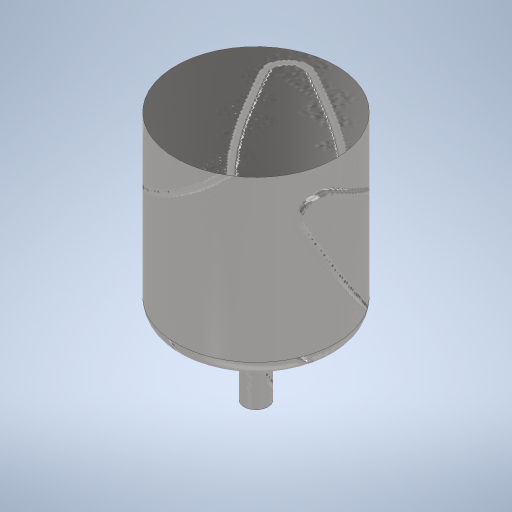
# Autodesk Inventor part: motor_ven
Saved by Autodesk Inventor 2023 (Build 270158000, 158)
## iProperties
Created: 2023-08-09
Part Number: motor_ven
Material: Genérico
Document SubType Name: Modeling
Designer: azeve
Density: 1 g/cm^3
Appearance: Padrão
Author: azeve
Autodesk Inventor part; units mm, degrees
ref_plane "YZ Plane" through (0, 0, 0) normal (1, 0, 0) x (0, 1, 0)
ref_plane "XZ Plane" through (0, 0, 0) normal (0, 1, 0) x (-1, 0, 0)
ref_plane "XY Plane" through (0, 0, 0) normal (0, 0, 1) x (1, 0, 0)
sketch "Esboço1" plane through (0, 0, 0) normal (0, 0, 1) x (1, 0, 0)
  line L0 (0, 0) -> (0, 22)
  line L1 (0, 22) -> (10, 22)
  line L2 (10, 22) -> (10, 19.8993)
  line L3 (10, 19.8993) -> (10, 0)
  line L4 (10, 0) -> (0, 0)
  line L5 (0, 0) -> (1.5, 0)
  line L6 (1.5, 0) -> (1.5, -9.13)
  line L7 (1.5, -9.13) -> (0, -9.13)
  line L8 (0, -9.13) -> (0, 0)
  line L9 (1.5, 0) -> (1.5, -1)
  line L10 (1.5, -1) -> (4.5, -1)
  line L11 (4.5, -1) -> (4.5, -6.8)
  line L12 (4.5, -6.8) -> (1.5, -6.8)
  line L13 (1.5, -6.8) -> (1.5, -1)
  line L14 (1.5, -6.8) -> (0, -6.8)
  line L15 (0, -1) -> (1.5, -1)
  line L16 (4.5, -1) -> (4.5, -3.025)
  line L17 (4.5, -3.025) -> (6.5557, -3.025)
  line L18 (6.5557, -3.025) -> (6.5557, -4.795)
  dimension "d0" = 22
  dimension "d1" = 10
  dimension "d2" = 1.5
  dimension "d4" = 9.13
  dimension "d7" = 1
  dimension "d8" = 3
  dimension "d9" = 5.8
  dimension "d10" = 2.025
  dimension "d11" = 1.77
  constraints: 38 end point, 8 point on line, 6 perpendicular, 5 vertical, 3 horizontal, 1 collinear
  measures "d0" distance of L0.start L0.end
  measures "d1" distance of L0.end L1.end
  measures "d2" distance of L0.start L5.end
  measures "d4" distance of L5.end L6.end
  measures "d7" distance of L5.end L9.end
  measures "d8" distance of L9.end L10.end
  measures "d9" distance of L10.end L11.end
  measures "d10" distance of L10.end L16.end
  measures "d11" distance of L17.end L18.end
revolve "Revolução1" add sketch "Esboço1" angle 360 about axis through (0, 0, 0) along (0, 1, 0) contours L0 L1 L2 L3 L4 | L4 L6 L15 L8 | L15 L6 L14 L8 | L14 L6 L7 L8
fillet "Arredondamento1" radius 2 1 edges at (-10, 0, 0)
